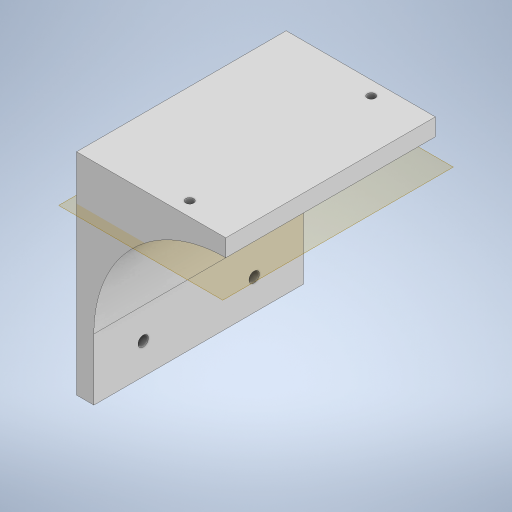
# Autodesk Inventor part: mainIMU
Saved by Autodesk Inventor 2024.2 (Build 282272000, 272)
## iProperties
Created: 2024-06-26
Part Number: mainIMU
Material: 一般
Document SubType Name: Modeling
Designer: towawa
Density: 1 g/cm^3
Appearance: 既定
Author: towawa
Autodesk Inventor part; units mm, degrees
ref_plane "YZ Plane" through (0, 0, 0) normal (1, 0, 0) x (0, 1, 0)
ref_plane "XZ Plane" through (0, 0, 0) normal (0, 1, 0) x (-1, 0, 0)
ref_plane "XY Plane" through (0, 0, 0) normal (0, 0, 1) x (1, 0, 0)
sketch "スケッチ1" plane through (0, 0, 0) normal (0, 0, 1) x (1, 0, 0)
  arc A0 (0, 53.5) -> (-53.5, 0) centre (0, 0) ccw
  line L0 (-60.5, 0) -> (-60.5, 60.5)
  line L1 (-60.5, 60.5) -> (0, 60.5)
  line L2 (0, 60.5) -> (0, -99.4363)
  line L3 (-60.5, 0) -> (-60.5, -25)
  line L4 (-60.5, -25) -> (-53.5, -25)
  line L5 (-53.5, -25) -> (-53.5, 0)
  dimension "d0" = 107
  dimension "d3" = 25
  constraints: 12 end point, 3 vertical, 2 point on circle, 1 centre point, 1 coincident, 1 horizontal, 1 perpendicular, 1 point on line
  measures "d0" diameter of A0
  measures "d3" distance of L0.start L3.end
extrude "押し出し1" add sketch "スケッチ1" along normal blind 85
sketch "スケッチ2" plane through (-60.5, 60.5, 0) normal (0, 1, 0) x (1, 0, 0)
  line L0 (60.5, -85) -> (7, -85) projected
  line L1 (60.5, -85) -> (60.5, -42.5)
  line L2 (60.5, 0) -> (60.5, -85) projected
  line L3 (60.5, -42.5) -> (40.18, -42.5)
  line L4 (40.18, -42.5) -> (40.18, -5.67)
  line L5 (40.18, -42.5) -> (40.18, -79.33)
  circle A0 centre (40.18, -5.67) radius 1.6
  circle A1 centre (40.18, -79.33) radius 1.6
  line L6 (60.5, -42.5) -> (-11.6627, -42.5)
  line L7 (-11.6627, -42.5) -> (-11.6627, -99.0684)
  line L8 (-11.6627, -99.0684) -> (60.5, -99.0684)
  line L9 (60.5, -99.0684) -> (60.5, -42.5)
  dimension "d8" = 20.32
  dimension "d9" = 36.83
  dimension "d10" = 36.83
  dimension "d11" = 3.2
  dimension "d12" = 3.2
  constraints: 16 end point, 2 centre point, 2 coincident, 2 horizontal, 2 parallel, 2 vertical, 1 midpoint, 1 perpendicular
  measures "d8" distance of L1.end L3.end
  measures "d9" distance of L3.end L4.end
  measures "d10" distance of L3.end L5.end
  measures "d11" diameter of A0
  measures "d12" diameter of A1
extrude "押し出し2" cut sketch "スケッチ2" against normal through all contours A0 | A1
ref_plane "作業平面1" through (-60.5, 42.25, 0) normal (0, 1, 0) x (1, 0, 0)
sketch "スケッチ3" plane through (-60.5, 42.25, 0) normal (0, 1, 0) x (1, 0, 0)
  circle A0 centre (40.18, -5.67) radius 1.6 projected
  line L0 (43.53, -5.67) -> (41.855, -8.5712)
  line L1 (41.855, -8.5712) -> (38.505, -8.5712)
  line L2 (38.505, -8.5712) -> (36.83, -5.67)
  line L3 (36.83, -5.67) -> (38.505, -2.7688)
  line L4 (38.505, -2.7688) -> (41.855, -2.7688)
  line L5 (41.855, -2.7688) -> (43.53, -5.67)
  point P0 (60.5, 0)
  dimension "d16" = 6.7
  constraints: 12 end point, 2 coincident, 13 other
  measures "d16" distance of L0.start L2.end
extrude "押し出し3" cut sketch "スケッチ3" along normal blind 11
extrude "押し出し4" cut sketch "スケッチ2" against normal through all contours L9 L8 L7 L6 L3 L1
mirror "ミラー1" about plane through (-72.1627, 60.5, 42.5) normal (0, 0, 1)
sketch "スケッチ4" plane through (-60.5, -25, 0) normal (-1, 0, 0) x (0, 0, 1)
  line L0 (85, 78.5) -> (0, 78.5) projected
  line L1 (0, 78.5) -> (85, 78.5)
  line L2 (85, 25) -> (0, 25) projected
  line L3 (0, 25) -> (85, 25)
  line L4 (0, 25) -> (0, 12.5)
  line L5 (0, 85.5) -> (0, 0) projected
  line L6 (0, 12.5) -> (85, 12.5)
  line L7 (85, 0) -> (85, 25) projected
  circle A0 centre (20, 12.5) radius 2.1
  line L8 (85, 12.5) -> (65, 12.5)
  circle A1 centre (65, 12.5) radius 2.1
  dimension "d21" = 12.5
  dimension "d22" = 4.2
  dimension "d23" = 20
  dimension "d24" = 20
  dimension "d25" = 4.2
  constraints: 10 end point, 3 point on line, 2 centre point, 2 collinear, 1 coincident, 1 midpoint
  measures "d21" distance of L2.end L4.end
  measures "d22" diameter of A0
  measures "d23" distance of L4.end A0.centre
  measures "d24" distance of L6.end L8.end
  measures "d25" diameter of A1
extrude "押し出し5" cut sketch "スケッチ4" against normal blind 10 contours A1 L6 | L6 A1 | A0 L6 | L6 A0
